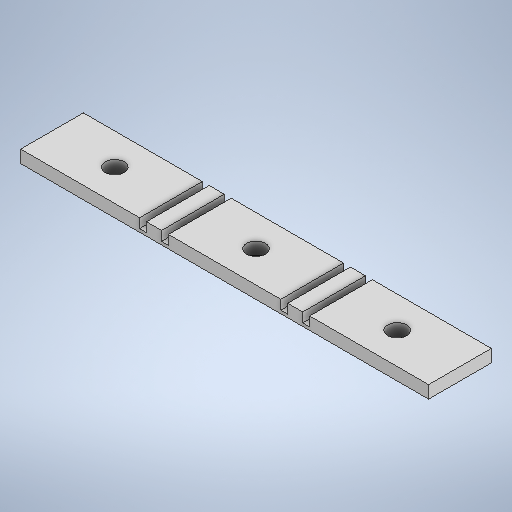
# Autodesk Inventor part: clamp
Saved by Autodesk Inventor 2025 (Build 290162000, 162)
## iProperties
Created: 2026-07-27
Part Number: clamp
Material: Generic
Document SubType Name: Modeling
Designer: DSTJOHN
Density: 1 g/cm^3
Appearance: Default
Author: DSTJOHN
Autodesk Inventor part; units mm, degrees
ref_plane "YZ Plane" through (0, 0, 0) normal (1, 0, 0) x (0, 1, 0)
ref_plane "XZ Plane" through (0, 0, 0) normal (0, 1, 0) x (-1, 0, 0)
ref_plane "XY Plane" through (0, 0, 0) normal (0, 0, 1) x (1, 0, 0)
sketch "Sketch1" plane through (0, 0, 0) normal (0, 1, 0) x (-1, 0, 0)
  line L0 (0, 0) -> (-130, 0)
  line L1 (-130, 0) -> (-130, -20)
  line L2 (-130, -20) -> (0, -20)
  line L3 (0, -20) -> (0, 0)
  line L4 (0, -10) -> (-130, -10) construction
  line L5 (-46, 0) -> (-46, -20) construction
  line L6 (-84, 0) -> (-84, -20) construction
  line L7 (-65, 0) -> (-65, -20) construction
  line L8 (-39, 0) -> (-39, -20) construction
  line L9 (-91, 0) -> (-91, -20) construction
  circle A0 centre (-65, -10) radius 3
  line L10 (-20, 0) -> (-20, -20) construction
  line L11 (-110, 0) -> (-110, -20) construction
  circle A1 centre (-110, -10) radius 3
  circle A2 centre (-20, -10) radius 3
  dimension "d1" = 20
  dimension "d0" = 130
  dimension "d2" = 65
  dimension "d3" = 26
  dimension "d4" = 26
  dimension "d5" = 19
  dimension "d6" = 19
  dimension "d17" = 6
  dimension "d18" = 20
  dimension "d19" = 20
  dimension "d20" = 6
  dimension "d21" = 6
  constraints: 20 end point, 8 vertical, 5 midpoint, 3 centre point, 1 parallel, 20 other
  measures "d0" distance between parallel lines of L1 L3
  measures "d2" distance between parallel lines of L7 L3
  measures "d3" distance between parallel lines of L7 L8
  measures "d4" distance between parallel lines of L9 L7
  measures "d5" distance between parallel lines of L7 L6
  measures "d6" distance between parallel lines of L7 L5
  measures "d17" diameter of A0
  measures "d18" distance between parallel lines of L10 L3
  measures "d19" distance between parallel lines of L1 L11
  measures "d20" diameter of A1
  measures "d21" diameter of A2
extrude "Extrusion1" add sketch "Sketch1" along normal blind 4
sketch "Sketch2" plane through (0, 4, 0) normal (0, 1, 0) x (1, 0, 0)
  line L0 (130, 20) -> (0, 20) construction
  line L1 (65, 20) -> (65, 0) construction
  line L2 (0, 0) -> (130, 0) construction
  line L3 (0, 20) -> (0, 0) construction
  line L4 (39, 20) -> (39, 0) construction
  line L5 (46, 20) -> (46, 0) construction
  line L6 (84, 20) -> (84, 0) construction
  line L7 (91, 20) -> (91, 0) construction
  line L8 (40.1, 20) -> (40.1, 0)
  line L9 (37.9, 20) -> (37.9, 0)
  line L10 (44.9, 20) -> (44.9, 0)
  line L11 (47.1, 20) -> (47.1, 0)
  line L12 (82.9, 20) -> (82.9, 0)
  line L13 (85.1, 20) -> (85.1, 0)
  line L14 (89.9, 20) -> (89.9, 0)
  line L15 (92.1, 20) -> (92.1, 0)
  line L16 (37.9, 20) -> (40.1, 20)
  line L17 (37.9, 0) -> (40.1, 0)
  line L18 (44.9, 0) -> (47.1, 0)
  line L19 (44.9, 20) -> (47.1, 20)
  line L20 (82.9, 20) -> (85.1, 20)
  line L21 (89.9, 20) -> (92.1, 20)
  line L22 (85.1, 0) -> (82.9, 0)
  line L23 (89.9, 0) -> (92.1, 0)
  dimension "d24" = 65
  dimension "d25" = 19
  dimension "d26" = 26
  dimension "d27" = 19
  dimension "d28" = 26
  dimension "d29" = 1.1
  dimension "d30" = 1.1
  dimension "d31" = 1.1
  dimension "d32" = 1.1
  dimension "d33" = 1.1
  dimension "d34" = 1.1
  dimension "d35" = 1.1
  dimension "d36" = 1.1
  constraints: 42 end point, 13 vertical, 6 horizontal, 2 perpendicular, 27 other
  measures "d24" distance between parallel lines of L1 L3
  measures "d25" distance between parallel lines of L1 L5
  measures "d26" distance between parallel lines of L1 L4
  measures "d27" distance between parallel lines of L6 L1
  measures "d28" distance between parallel lines of L1 L7
  measures "d29" distance between parallel lines of L4 L9
  measures "d30" distance between parallel lines of L8 L4
  measures "d31" distance between parallel lines of L5 L10
  measures "d32" distance between parallel lines of L11 L5
  measures "d33" distance between parallel lines of L6 L12
  measures "d34" distance between parallel lines of L13 L6
  measures "d35" distance between parallel lines of L7 L14
  measures "d36" distance between parallel lines of L15 L7
extrude "Extrusion2" cut sketch "Sketch2" against normal blind 3
body "Solid1"
